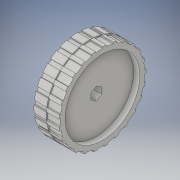
# Autodesk Inventor part: WheelV2
Saved by Autodesk Inventor 2019 (Build 230136000, 136)
## iProperties
Created: 2021-09-16
Part Number: WheelV2
Material: Generic
Document SubType Name: Modeling
Designer: timmy
Density: 1 g/cm^3
Appearance: Default
Author: timmy
Autodesk Inventor part; units mm, degrees
ref_plane "YZ Plane" through (0, 0, 0) normal (1, 0, 0) x (0, 1, 0)
ref_plane "XZ Plane" through (0, 0, 0) normal (0, 1, 0) x (-1, 0, 0)
sketch "Sketch1" plane through (0, 0, 0) normal (1, 0, 0) x (0, 1, 0)
  circle A0 centre (0, 0) radius 83.82
  circle A1 centre (0, 0) radius 86.36 construction
  line L0 (86.36, 0) -> (86.0238, -7.6126)
  line L1 (86.0238, -7.6126) -> (88.5638, -7.7247)
  line L2 (86.36, 0) -> (88.9, 0)
  line L3 (83.6468, 21.4769) -> (86.107, 22.1085)
  line L4 (83.6468, 21.4769) -> (85.2144, 14.0198)
  line L5 (85.2144, 14.0198) -> (87.7024, 14.5429)
  line L6 (75.6778, 41.6042) -> (77.9037, 42.8279)
  line L7 (75.6778, 41.6042) -> (79.0506, 34.7713)
  line L8 (79.0506, 34.7713) -> (81.3304, 35.8967)
  line L9 (62.9537, 59.1175) -> (64.8053, 60.8562)
  line L10 (62.9537, 59.1175) -> (67.9198, 53.338)
  line L11 (67.9198, 53.338) -> (69.8481, 54.995)
  line L12 (46.274, 72.9162) -> (47.635, 75.0608)
  line L13 (46.274, 72.9162) -> (52.5214, 68.5533)
  line L14 (52.5214, 68.5533) -> (53.9771, 70.6377)
  line L15 (26.6867, 82.1332) -> (27.4716, 84.5489)
  line L16 (26.6867, 82.1332) -> (33.8228, 79.4611)
  line L17 (33.8228, 79.4611) -> (34.7144, 81.8421)
  line L18 (5.4226, 86.1896) -> (5.5821, 88.7246)
  line L19 (5.4226, 86.1896) -> (12.999, 85.3761)
  line L20 (12.999, 85.3761) -> (13.2705, 87.904)
  line L21 (-16.1823, 84.8303) -> (-16.6582, 87.3253)
  line L22 (-16.1823, 84.8303) -> (-8.6415, 85.9266)
  line L23 (-8.6415, 85.9266) -> (-9.0073, 88.4425)
  line L24 (-36.7703, 78.1409) -> (-37.8518, 80.4391)
  line L25 (-36.7703, 78.1409) -> (-29.7391, 81.078)
  line L26 (-29.7391, 81.078) -> (-30.7191, 83.4239)
  line L27 (-55.0479, 66.5415) -> (-56.667, 68.4986)
  line L28 (-55.0479, 66.5415) -> (-48.9681, 71.1349)
  line L29 (-48.9681, 71.1349) -> (-50.5006, 73.1635)
  line L30 (-69.8667, 50.7611) -> (-71.9216, 52.2541)
  line L31 (-69.8667, 50.7611) -> (-65.1202, 56.7222)
  line L32 (-65.1202, 56.7222) -> (-67.1091, 58.3059)
  line L33 (-80.2955, 31.7912) -> (-82.6571, 32.7263)
  line L34 (-80.2955, 31.7912) -> (-77.1806, 38.7455)
  line L35 (-77.1806, 38.7455) -> (-79.5008, 39.7848)
  line L36 (-85.679, 10.8238) -> (-88.199, 11.1421)
  line L37 (-85.679, 10.8238) -> (-84.3914, 18.3342)
  line L38 (-84.3914, 18.3342) -> (-86.8972, 18.7638)
  line L39 (-85.679, -10.8238) -> (-88.199, -11.1421)
  line L40 (-85.679, -10.8238) -> (-86.2996, -3.2291)
  line L41 (-86.2996, -3.2291) -> (-88.8336, -3.4361)
  line L42 (-80.2955, -31.7912) -> (-82.6571, -32.7263)
  line L43 (-80.2955, -31.7912) -> (-82.7853, -24.5895)
  line L44 (-82.7853, -24.5895) -> (-85.1882, -25.4202)
  line L45 (-69.8667, -50.7611) -> (-71.9216, -52.2541)
  line L46 (-69.8667, -50.7611) -> (-74.0693, -44.4048)
  line L47 (-74.0693, -44.4048) -> (-76.1901, -45.807)
  line L48 (-55.0479, -66.5415) -> (-56.667, -68.4986)
  line L49 (-55.0479, -66.5415) -> (-60.6992, -61.4301)
  line L50 (-60.6992, -61.4301) -> (-62.4047, -63.3156)
  line L51 (-36.7703, -78.1409) -> (-37.8518, -80.4391)
  line L52 (-36.7703, -78.1409) -> (-43.5152, -74.5954)
  line L53 (-43.5152, -74.5954) -> (-44.6982, -76.8458)
  line L54 (-16.1823, -84.8303) -> (-16.6582, -87.3253)
  line L55 (-16.1823, -84.8303) -> (-23.597, -83.0736)
  line L56 (-23.597, -83.0736) -> (-24.1831, -85.5476)
  line L57 (5.4226, -86.1896) -> (5.5821, -88.7246)
  line L58 (5.4226, -86.1896) -> (-2.1961, -86.3321)
  line L59 (-2.1961, -86.3321) -> (-2.1485, -88.874)
  line L60 (26.6867, -82.1332) -> (27.4716, -84.5489)
  line L61 (26.6867, -82.1332) -> (19.3428, -84.1659)
  line L62 (19.3428, -84.1659) -> (20.021, -86.6162)
  line L63 (46.274, -72.9162) -> (47.635, -75.0608)
  line L64 (46.274, -72.9162) -> (39.6664, -76.7113)
  line L65 (39.6664, -76.7113) -> (40.9326, -78.916)
  line L66 (62.9537, -59.1175) -> (64.8053, -60.8562)
  line L67 (62.9537, -59.1175) -> (57.4975, -64.4367)
  line L68 (57.4975, -64.4367) -> (59.2722, -66.2572)
  line L69 (75.6778, -41.6042) -> (77.9037, -42.8279)
  line L70 (75.6778, -41.6042) -> (71.7159, -48.1132)
  line L71 (71.7159, -48.1132) -> (73.8876, -49.4352)
  line L72 (83.6468, -21.4769) -> (86.107, -22.1085)
  line L73 (83.6468, -21.4769) -> (81.4281, -28.7667)
  line L74 (81.4281, -28.7667) -> (83.8603, -29.507)
  arc A2 (86.107, 22.1085) -> (81.3304, 35.8967) centre (0, 0) ccw
  arc A3 (88.9, 0) -> (87.7024, 14.5429) centre (0, 0) ccw
  arc A4 (86.107, -22.1085) -> (88.5638, -7.7247) centre (0, 0) ccw
  arc A5 (77.9037, -42.8279) -> (83.8603, -29.507) centre (0, 0) ccw
  arc A6 (64.8053, -60.8562) -> (73.8876, -49.4352) centre (0, 0) ccw
  arc A7 (47.635, -75.0608) -> (59.2722, -66.2572) centre (0, 0) ccw
  arc A8 (27.4716, -84.5489) -> (40.9326, -78.916) centre (0, 0) ccw
  arc A9 (77.9037, 42.8279) -> (69.8481, 54.995) centre (0, 0) ccw
  arc A10 (64.8053, 60.8562) -> (53.9771, 70.6377) centre (0, 0) ccw
  arc A11 (47.635, 75.0608) -> (34.7144, 81.8421) centre (0, 0) ccw
  arc A12 (27.4716, 84.5489) -> (13.2705, 87.904) centre (0, 0) ccw
  arc A13 (5.5821, 88.7246) -> (-9.0073, 88.4425) centre (0, 0) ccw
  arc A14 (-16.6582, 87.3253) -> (-30.7191, 83.4239) centre (0, 0) ccw
  arc A15 (-37.8518, 80.4391) -> (-50.5006, 73.1635) centre (0, 0) ccw
  arc A16 (-56.667, 68.4986) -> (-67.1091, 58.3059) centre (0, 0) ccw
  arc A17 (-71.9216, 52.2541) -> (-79.5008, 39.7848) centre (0, 0) ccw
  arc A18 (-82.6571, 32.7263) -> (-86.8972, 18.7638) centre (0, 0) ccw
  arc A19 (-88.199, 11.1421) -> (-88.8336, -3.4361) centre (0, 0) ccw
  arc A20 (-88.199, -11.1421) -> (-85.1882, -25.4202) centre (0, 0) ccw
  arc A21 (-82.6571, -32.7263) -> (-76.1901, -45.807) centre (0, 0) ccw
  arc A22 (-71.9216, -52.2541) -> (-62.4047, -63.3156) centre (0, 0) ccw
  arc A23 (-56.667, -68.4986) -> (-44.6982, -76.8458) centre (0, 0) ccw
  arc A24 (-37.8518, -80.4391) -> (-24.1831, -85.5476) centre (0, 0) ccw
  arc A25 (-16.6582, -87.3253) -> (-2.1485, -88.874) centre (0, 0) ccw
  arc A26 (5.5821, -88.7246) -> (20.021, -86.6162) centre (0, 0) ccw
  dimension "d14" = 7.62
  dimension "d17" = 360
  constraints: 150 end point, 50 point on circle, 26 centre point, 1 coincident, 1 horizontal, 1 perpendicular, 179 other
  measures "d14" distance of L0.start L0.end
extrude "Extrusion1" add sketch "Sketch1" along normal blind 50.8 contours A0 | L0 L1 A4 L72 L73 L74 A5 L69 L70 L71 A6 L66 L67 L68 A7 L63 L64 L65 A8 L60 L61 L62 A26 L57 L58 L59 A25 L54 L55 L56 A24 L51 L52 L53 A23 L48 L49 L50 A22 L45 L46 L47 A21 L42 L43 L44 A20 L39 L40 L41 A19 L36 L37 L38 A18 L33 L34 L35 A17 L30 L31 L32 A16 L27 L28 L29 A15 L24 L25 L26 A14 L21 L22 L23 A13 L18 L19 L20 A12 L15 L16 L17 A11 L12 L13 L14 A10 L9 L10 L11 A9 L6 L7 L8 A2 L3 L4 L5 A3 L2
sketch "Sketch2" plane through (50.8, 0, 0) normal (1, 0, 0) x (0, -0.3273, 0.9449)
  arc A0 (-7.296, -88.6001) -> (7.296, -88.6001) centre (0, 0) ccw projected
  circle A1 centre (0, 0) radius 76.2
  line L0 (-35.3524, -78.7925) -> (-28.2693, -81.6021) projected
  line L1 (-28.2693, -81.6021) -> (-29.1008, -84.0021) projected
  arc A2 (-29.1008, -84.0021) -> (-14.9671, -87.631) centre (0, 0) ccw projected
  line L2 (-14.9671, -87.631) -> (-14.6469, -85.1089) projected
  line L3 (-14.6469, -85.1089) -> (-7.0876, -86.0687) projected
  line L4 (-7.0876, -86.0687) -> (-7.296, -88.6001) projected
  line L5 (7.296, -88.6001) -> (6.979, -86.0775) projected
  line L6 (6.979, -86.0775) -> (14.5395, -85.1273) projected
  line L7 (14.5395, -85.1273) -> (14.9671, -87.631) projected
  arc A3 (14.9671, -87.631) -> (29.1008, -84.0021) centre (0, 0) ccw projected
  line L8 (29.1008, -84.0021) -> (28.1663, -81.6377) projected
  line L9 (28.1663, -81.6377) -> (35.253, -78.837) projected
  line L10 (35.253, -78.837) -> (36.2899, -81.1558) projected
  arc A4 (36.2899, -81.1558) -> (49.077, -74.126) centre (0, 0) ccw projected
  line L11 (49.077, -74.126) -> (47.5839, -72.0682) projected
  line L12 (47.5839, -72.0682) -> (53.7514, -67.5931) projected
  line L13 (53.7514, -67.5931) -> (55.3324, -69.5812) projected
  arc A5 (55.3324, -69.5812) -> (65.9695, -59.5922) centre (0, 0) ccw projected
  line L14 (65.9695, -59.5922) -> (64.0116, -57.9704) projected
  line L15 (64.0116, -57.9704) -> (68.8725, -52.1021) projected
  line L16 (68.8725, -52.1021) -> (70.8981, -53.6346) projected
  arc A6 (70.8981, -53.6346) -> (78.717, -41.3141) centre (0, 0) ccw projected
  line L17 (78.717, -41.3141) -> (76.4172, -40.2301) projected
  line L18 (76.4172, -40.2301) -> (79.666, -33.3374) projected
  line L19 (79.666, -33.3374) -> (82.0091, -34.3179) projected
  arc A7 (82.0091, -34.3179) -> (86.5183, -20.44) centre (0, 0) ccw projected
  line L20 (86.5183, -20.44) -> (84.0212, -19.962) projected
  line L21 (84.0212, -19.962) -> (85.4538, -12.4779) projected
  line L22 (85.4538, -12.4779) -> (87.9671, -12.8449) projected
  arc A8 (87.9671, -12.8449) -> (88.8834, 1.7184) centre (0, 0) ccw projected
  line L23 (88.8834, 1.7184) -> (86.3459, 1.5604) projected
  line L24 (86.3459, 1.5604) -> (85.8722, 9.1656) projected
  line L25 (85.8722, 9.1656) -> (88.3979, 9.4352) projected
  arc A9 (88.3979, 9.4352) -> (85.6636, 23.7688) centre (0, 0) ccw projected
  line L26 (85.6636, 23.7688) -> (83.2451, 22.9847) projected
  line L27 (83.2451, 22.9847) -> (80.895, 30.2332) projected
  line L28 (80.895, 30.2332) -> (83.2743, 31.1224) projected
  arc A10 (83.2743, 31.1224) -> (77.0613, 44.3257) centre (0, 0) ccw projected
  line L29 (77.0613, 44.3257) -> (74.9138, 42.9648) projected
  line L30 (74.9138, 42.9648) -> (70.8348, 49.4012) projected
  line L31 (70.8348, 49.4012) -> (72.9182, 50.8541) projected
  arc A11 (72.9182, 50.8541) -> (63.6169, 62.0975) centre (0, 0) ccw projected
  line L32 (63.6169, 62.0975) -> (61.8753, 60.2453) projected
  line L33 (61.8753, 60.2453) -> (56.3239, 65.465) projected
  line L34 (56.3239, 65.465) -> (57.9805, 67.3905) projected
  arc A12 (57.9805, 67.3905) -> (46.1752, 75.9675) centre (0, 0) ccw projected
  line L35 (46.1752, 75.9675) -> (44.949, 73.7403) projected
  line L36 (44.949, 73.7403) -> (38.2739, 77.4155) projected
  line L37 (38.2739, 77.4155) -> (39.3996, 79.6924) projected
  arc A13 (39.3996, 79.6924) -> (25.8322, 85.0641) centre (0, 0) ccw projected
  line L38 (25.8322, 85.0641) -> (25.1984, 82.602) projected
  line L39 (25.1984, 82.602) -> (17.819, 84.5017) projected
  line L40 (17.819, 84.5017) -> (18.343, 86.987) projected
  arc A14 (18.343, 86.987) -> (3.866, 88.8159) centre (0, 0) ccw projected
  line L41 (3.866, 88.8159) -> (3.8644, 86.2735) projected
  line L42 (3.8644, 86.2735) -> (-3.7556, 86.2783) projected
  line L43 (-3.7556, 86.2783) -> (-3.866, 88.8159) projected
  arc A15 (-3.866, 88.8159) -> (-18.343, 86.987) centre (0, 0) ccw projected
  line L44 (-18.343, 86.987) -> (-17.7123, 84.5241) projected
  line L45 (-17.7123, 84.5241) -> (-25.0941, 82.6337) projected
  line L46 (-25.0941, 82.6337) -> (-25.8322, 85.0641) projected
  arc A16 (-25.8322, 85.0641) -> (-39.3996, 79.6924) centre (0, 0) ccw projected
  line L47 (-39.3996, 79.6924) -> (-38.1762, 77.4637) projected
  line L48 (-38.1762, 77.4637) -> (-44.8559, 73.797) projected
  line L49 (-44.8559, 73.797) -> (-46.1752, 75.9675) projected
  arc A17 (-46.1752, 75.9675) -> (-57.9805, 67.3905) centre (0, 0) ccw projected
  line L50 (-57.9805, 67.3905) -> (-56.2412, 65.5361) projected
  line L51 (-56.2412, 65.5361) -> (-61.7993, 60.3233) projected
  line L52 (-61.7993, 60.3233) -> (-63.6169, 62.0975) projected
  arc A18 (-63.6169, 62.0975) -> (-72.9182, 50.8541) centre (0, 0) ccw projected
  line L53 (-72.9182, 50.8541) -> (-70.7725, 49.4905) projected
  line L54 (-70.7725, 49.4905) -> (-74.8595, 43.0593) projected
  line L55 (-74.8595, 43.0593) -> (-77.0613, 44.3257) projected
  arc A19 (-77.0613, 44.3257) -> (-83.2743, 31.1224) centre (0, 0) ccw projected
  line L56 (-83.2743, 31.1224) -> (-80.8568, 30.3353) projected
  line L57 (-80.8568, 30.3353) -> (-83.2161, 23.0897) projected
  line L58 (-83.2161, 23.0897) -> (-85.6636, 23.7688) projected
  arc A20 (-85.6636, 23.7688) -> (-88.3979, 9.4352) centre (0, 0) ccw projected
  line L59 (-88.3979, 9.4352) -> (-85.8606, 9.274) projected
  line L60 (-85.8606, 9.274) -> (-86.3439, 1.6693) projected
  line L61 (-86.3439, 1.6693) -> (-88.8834, 1.7184) projected
  arc A21 (-88.8834, 1.7184) -> (-87.9671, -12.8449) centre (0, 0) ccw projected
  line L62 (-87.9671, -12.8449) -> (-85.4695, -12.3701) projected
  line L63 (-85.4695, -12.3701) -> (-84.0464, -19.856) projected
  line L64 (-84.0464, -19.856) -> (-86.5183, -20.44) projected
  arc A22 (-86.5183, -20.44) -> (-82.0091, -34.3179) centre (0, 0) ccw projected
  line L65 (-82.0091, -34.3179) -> (-79.708, -33.2368) projected
  line L66 (-79.708, -33.2368) -> (-76.4679, -40.1337) projected
  line L67 (-76.4679, -40.1337) -> (-78.717, -41.3141) projected
  arc A23 (-78.717, -41.3141) -> (-70.8981, -53.6346) centre (0, 0) ccw projected
  line L68 (-70.8981, -53.6346) -> (-68.9381, -52.0152) projected
  line L69 (-68.9381, -52.0152) -> (-64.0847, -57.8896) projected
  line L70 (-64.0847, -57.8896) -> (-65.9695, -59.5922) projected
  arc A24 (-65.9695, -59.5922) -> (-55.3324, -69.5812) centre (0, 0) ccw projected
  line L71 (-55.3324, -69.5812) -> (-53.8367, -67.5253) projected
  line L72 (-53.8367, -67.5253) -> (-47.6748, -72.0081) projected
  line L73 (-47.6748, -72.0081) -> (-49.077, -74.126) projected
  arc A25 (-49.077, -74.126) -> (-36.2899, -81.1558) centre (0, 0) ccw projected
  line L74 (-36.2899, -81.1558) -> (-35.3524, -78.7925) projected
  dimension "d3" = 12.7
  constraints: 1 centre point
  measures "d3" radial gap between concentric circles of A0 A1
extrude "Extrusion2" cut sketch "Sketch2" against normal blind 12.7 contours A1
sketch "Sketch4" plane through (0, 0, 0) normal (-1, 0, 0) x (0, 0.3273, -0.9449)
  circle A0 centre (0, 0) radius 76.2 projected
extrude "Extrusion3" cut sketch "Sketch4" against normal blind 12.7
sketch "Sketch5" plane through (38.1, 0, 0) normal (1, 0, 0) x (0, 0, -1)
  line L0 (0, 0) -> (0, 12.7)
  line L1 (0, 12.7) -> (10.9985, 6.35)
  line L2 (10.9985, 6.35) -> (10.9985, -6.35)
  line L3 (10.9985, -6.35) -> (0, -12.7)
  line L4 (0, -12.7) -> (-10.9985, -6.35)
  line L5 (-10.9985, -6.35) -> (-10.9985, 6.35)
  line L6 (-10.9985, 6.35) -> (0, 12.7)
  dimension "d8" = 12.7
  constraints: 14 end point, 1 coincident, 1 vertical, 13 other
  measures "d8" distance of L0.start L0.end
extrude "Extrusion4" cut sketch "Sketch5" against normal blind 127
ref_plane "Work Plane1" through (25.4, 0, 0) normal (1, 0, 0) x (0, 0, -1)
sketch "Sketch6" plane through (25.4, 0, 0) normal (1, 0, 0) x (0, 0, -1)
  circle A0 centre (0, 0) radius 76.2 projected
  line L0 (7.6126, 86.0238) -> (0, 86.36) projected
  line L1 (0, 86.36) -> (0, 88.9) projected
  arc A1 (0, 88.9) -> (-14.5429, 87.7024) centre (0, 0) ccw projected
  line L2 (-14.5429, 87.7024) -> (-14.0198, 85.2144) projected
  line L3 (-14.0198, 85.2144) -> (-21.4769, 83.6468) projected
  line L4 (-21.4769, 83.6468) -> (-22.1085, 86.107) projected
  arc A2 (-22.1085, 86.107) -> (-35.8967, 81.3304) centre (0, 0) ccw projected
  line L5 (-35.8967, 81.3304) -> (-34.7713, 79.0506) projected
  line L6 (-34.7713, 79.0506) -> (-41.6042, 75.6778) projected
  line L7 (-41.6042, 75.6778) -> (-42.8279, 77.9037) projected
  arc A3 (-42.8279, 77.9037) -> (-54.995, 69.8481) centre (0, 0) ccw projected
  line L8 (-54.995, 69.8481) -> (-53.338, 67.9198) projected
  line L9 (-53.338, 67.9198) -> (-59.1175, 62.9537) projected
  line L10 (-59.1175, 62.9537) -> (-60.8562, 64.8053) projected
  arc A4 (-60.8562, 64.8053) -> (-70.6377, 53.9771) centre (0, 0) ccw projected
  line L11 (-70.6377, 53.9771) -> (-68.5533, 52.5214) projected
  line L12 (-68.5533, 52.5214) -> (-72.9162, 46.274) projected
  line L13 (-72.9162, 46.274) -> (-75.0608, 47.635) projected
  arc A5 (-75.0608, 47.635) -> (-81.8421, 34.7144) centre (0, 0) ccw projected
  line L14 (-81.8421, 34.7144) -> (-79.4611, 33.8228) projected
  line L15 (-79.4611, 33.8228) -> (-82.1332, 26.6867) projected
  line L16 (-82.1332, 26.6867) -> (-84.5489, 27.4716) projected
  arc A6 (-84.5489, 27.4716) -> (-87.904, 13.2705) centre (0, 0) ccw projected
  line L17 (-87.904, 13.2705) -> (-85.3761, 12.999) projected
  line L18 (-85.3761, 12.999) -> (-86.1896, 5.4226) projected
  line L19 (-86.1896, 5.4226) -> (-88.7246, 5.5821) projected
  arc A7 (-88.7246, 5.5821) -> (-88.4425, -9.0073) centre (0, 0) ccw projected
  line L20 (-88.4425, -9.0073) -> (-85.9266, -8.6415) projected
  line L21 (-85.9266, -8.6415) -> (-84.8303, -16.1823) projected
  line L22 (-84.8303, -16.1823) -> (-87.3253, -16.6582) projected
  arc A8 (-87.3253, -16.6582) -> (-83.4239, -30.7191) centre (0, 0) ccw projected
  line L23 (-83.4239, -30.7191) -> (-81.078, -29.7391) projected
  line L24 (-81.078, -29.7391) -> (-78.1409, -36.7703) projected
  line L25 (-78.1409, -36.7703) -> (-80.4391, -37.8518) projected
  arc A9 (-80.4391, -37.8518) -> (-73.1635, -50.5006) centre (0, 0) ccw projected
  line L26 (-73.1635, -50.5006) -> (-71.1349, -48.9681) projected
  line L27 (-71.1349, -48.9681) -> (-66.5415, -55.0479) projected
  line L28 (-66.5415, -55.0479) -> (-68.4986, -56.667) projected
  arc A10 (-68.4986, -56.667) -> (-58.3059, -67.1091) centre (0, 0) ccw projected
  line L29 (-58.3059, -67.1091) -> (-56.7222, -65.1202) projected
  line L30 (-56.7222, -65.1202) -> (-50.7611, -69.8667) projected
  line L31 (-50.7611, -69.8667) -> (-52.2541, -71.9216) projected
  arc A11 (-52.2541, -71.9216) -> (-39.7848, -79.5008) centre (0, 0) ccw projected
  line L32 (-39.7848, -79.5008) -> (-38.7455, -77.1806) projected
  line L33 (-38.7455, -77.1806) -> (-31.7912, -80.2955) projected
  line L34 (-31.7912, -80.2955) -> (-32.7263, -82.6571) projected
  arc A12 (-32.7263, -82.6571) -> (-18.7638, -86.8972) centre (0, 0) ccw projected
  line L35 (-18.7638, -86.8972) -> (-18.3342, -84.3914) projected
  line L36 (-18.3342, -84.3914) -> (-10.8238, -85.679) projected
  line L37 (-10.8238, -85.679) -> (-11.1421, -88.199) projected
  arc A13 (-11.1421, -88.199) -> (3.4361, -88.8336) centre (0, 0) ccw projected
  line L38 (3.4361, -88.8336) -> (3.2291, -86.2996) projected
  line L39 (3.2291, -86.2996) -> (10.8238, -85.679) projected
  line L40 (10.8238, -85.679) -> (11.1421, -88.199) projected
  arc A14 (11.1421, -88.199) -> (25.4202, -85.1882) centre (0, 0) ccw projected
  line L41 (25.4202, -85.1882) -> (24.5895, -82.7853) projected
  line L42 (24.5895, -82.7853) -> (31.7912, -80.2955) projected
  line L43 (31.7912, -80.2955) -> (32.7263, -82.6571) projected
  arc A15 (32.7263, -82.6571) -> (45.807, -76.1901) centre (0, 0) ccw projected
  line L44 (45.807, -76.1901) -> (44.4048, -74.0693) projected
  line L45 (44.4048, -74.0693) -> (50.7611, -69.8667) projected
  line L46 (50.7611, -69.8667) -> (52.2541, -71.9216) projected
  arc A16 (52.2541, -71.9216) -> (63.3156, -62.4047) centre (0, 0) ccw projected
  line L47 (63.3156, -62.4047) -> (61.4301, -60.6992) projected
  line L48 (61.4301, -60.6992) -> (66.5415, -55.0479) projected
  line L49 (66.5415, -55.0479) -> (68.4986, -56.667) projected
  arc A17 (68.4986, -56.667) -> (76.8458, -44.6982) centre (0, 0) ccw projected
  line L50 (76.8458, -44.6982) -> (74.5954, -43.5152) projected
  line L51 (74.5954, -43.5152) -> (78.1409, -36.7703) projected
  line L52 (78.1409, -36.7703) -> (80.4391, -37.8518) projected
  arc A18 (80.4391, -37.8518) -> (85.5476, -24.1831) centre (0, 0) ccw projected
  line L53 (85.5476, -24.1831) -> (83.0736, -23.597) projected
  line L54 (83.0736, -23.597) -> (84.8303, -16.1823) projected
  line L55 (84.8303, -16.1823) -> (87.3253, -16.6582) projected
  arc A19 (87.3253, -16.6582) -> (88.874, -2.1485) centre (0, 0) ccw projected
  line L56 (88.874, -2.1485) -> (86.3321, -2.1961) projected
  line L57 (86.3321, -2.1961) -> (86.1896, 5.4226) projected
  line L58 (86.1896, 5.4226) -> (88.7246, 5.5821) projected
  arc A20 (88.7246, 5.5821) -> (86.6162, 20.021) centre (0, 0) ccw projected
  line L59 (86.6162, 20.021) -> (84.1659, 19.3428) projected
  line L60 (84.1659, 19.3428) -> (82.1332, 26.6867) projected
  line L61 (82.1332, 26.6867) -> (84.5489, 27.4716) projected
  arc A21 (84.5489, 27.4716) -> (78.916, 40.9326) centre (0, 0) ccw projected
  line L62 (78.916, 40.9326) -> (76.7113, 39.6664) projected
  line L63 (76.7113, 39.6664) -> (72.9162, 46.274) projected
  line L64 (72.9162, 46.274) -> (75.0608, 47.635) projected
  arc A22 (75.0608, 47.635) -> (66.2572, 59.2722) centre (0, 0) ccw projected
  line L65 (66.2572, 59.2722) -> (64.4367, 57.4975) projected
  line L66 (64.4367, 57.4975) -> (59.1175, 62.9537) projected
  line L67 (59.1175, 62.9537) -> (60.8562, 64.8053) projected
  arc A23 (60.8562, 64.8053) -> (49.4352, 73.8876) centre (0, 0) ccw projected
  line L68 (49.4352, 73.8876) -> (48.1132, 71.7159) projected
  line L69 (48.1132, 71.7159) -> (41.6042, 75.6778) projected
  line L70 (41.6042, 75.6778) -> (42.8279, 77.9037) projected
  arc A24 (42.8279, 77.9037) -> (29.507, 83.8603) centre (0, 0) ccw projected
  line L71 (29.507, 83.8603) -> (28.7667, 81.4281) projected
  line L72 (28.7667, 81.4281) -> (21.4769, 83.6468) projected
  line L73 (21.4769, 83.6468) -> (22.1085, 86.107) projected
  arc A25 (22.1085, 86.107) -> (7.7247, 88.5638) centre (0, 0) ccw projected
  line L74 (7.7247, 88.5638) -> (7.6126, 86.0238) projected
  line L75 (-60.8562, 64.8053) -> (-59.1175, 62.9537) projected
  line L76 (-60.8562, 64.8053) -> (-54.995, 69.8481)
  line L77 (-35.8967, 81.3304) -> (-34.7713, 79.0506) projected
  line L78 (-42.8279, 77.9037) -> (-35.8967, 81.3304)
  line L79 (-35.8967, 81.3304) -> (-22.1085, 86.107)
  line L80 (-14.0198, 85.2144) -> (-14.5429, 87.7024) projected
  line L81 (-14.5429, 87.7024) -> (-22.1085, 86.107)
  line L82 (0, 88.9) -> (7.7247, 88.5638)
  line L83 (22.1085, 86.107) -> (29.507, 83.8603)
  line L84 (42.8279, 77.9037) -> (49.4352, 73.8876)
  line L85 (60.8562, 64.8053) -> (66.2572, 59.2722)
  line L86 (78.916, 40.9326) -> (75.0608, 47.635)
  line L87 (84.5489, 27.4716) -> (86.6162, 20.021)
  line L88 (88.874, -2.1485) -> (88.7246, 5.5821)
  line L89 (-75.0608, 47.635) -> (-70.6377, 53.9771)
  line L90 (-84.5489, 27.4716) -> (-81.8421, 34.7144)
  line L91 (-87.904, 13.2705) -> (-85.3761, 12.999) projected
  line L92 (-88.7246, 5.5821) -> (-87.904, 13.2705)
  arc A26 (-84.5489, 27.4716) -> (-87.904, 13.2705) centre (0, 0) ccw projected
  arc A27 (-87.3253, -16.6582) -> (-83.4239, -30.7191) centre (0, 0) ccw projected
  line L93 (-87.3253, -16.6582) -> (-88.4425, -9.0073)
  line L94 (-83.4239, -30.7191) -> (-80.4391, -37.8518)
  arc A28 (-68.4986, -56.667) -> (-58.3059, -67.1091) centre (0, 0) ccw projected
  line L95 (-73.1635, -50.5006) -> (-68.4986, -56.667)
  line L96 (-58.3059, -67.1091) -> (-52.2541, -71.9216)
  arc A29 (-52.2541, -71.9216) -> (-39.7848, -79.5008) centre (0, 0) ccw projected
  line L97 (-39.7848, -79.5008) -> (-32.7263, -82.6571)
  line L98 (-18.7638, -86.8972) -> (-11.1421, -88.199)
  line L99 (3.4361, -88.8336) -> (11.1421, -88.199)
  line L100 (25.4202, -85.1882) -> (32.7263, -82.6571)
  line L101 (52.2541, -71.9216) -> (45.807, -76.1901)
  line L102 (63.3156, -62.4047) -> (68.4986, -56.667)
  line L103 (80.4391, -37.8518) -> (76.8458, -44.6982)
  line L104 (87.3253, -16.6582) -> (85.5476, -24.1831)
  constraints: 52 end point
extrude "Extrusion5" add sketch "Sketch6" along normal up to surface (25.4 mm away) contours L0 L1 L82 L74 | L83 L71 L72 L73 | L2 L3 L4 L81 | L84 L68 L69 L70 | L5 L6 L7 L78 | L85 L65 L66 L67 | L8 L9 L10 L76 | L86 L62 L63 L64 | L11 L12 L13 L89 | L87 L59 L60 L61 | L14 L15 L16 L90 | L88 L56 L57 L58 | L17 L18 L19 L92 | L104 L53 L54 L55 | L20 L21 L22 L93 | L103 L50 L51 L52 | L23 L24 L25 L94 | L102 L47 L48 L49 | L26 L27 L28 L95 | L101 L44 L45 L46 | L29 L30 L31 L96 | L100 L41 L42 L43 | L32 L33 L34 L97 | L99 L38 L39 L40 | L35 L36 L37 L98
sketch "Sketch7" plane through (50.8, 0, 0) normal (1, 0, 0) x (0, 0, -1)
  line L0 (22.1085, 86.107) -> (29.507, 83.8603) projected
  line L1 (0, 88.9) -> (7.7247, 88.5638) projected
  line L2 (-75.0608, 47.635) -> (-70.6377, 53.9771) projected
  line L3 (-84.5489, 27.4716) -> (-81.8421, 34.7144) projected
  line L4 (-88.7246, 5.5821) -> (-87.904, 13.2705) projected
  line L5 (-87.3253, -16.6582) -> (-88.4425, -9.0073) projected
  line L6 (-80.4391, -37.8518) -> (-83.4239, -30.7191) projected
  line L7 (42.8279, 77.9037) -> (49.4352, 73.8876) projected
  line L8 (60.8562, 64.8053) -> (66.2572, 59.2722) projected
  line L9 (75.0608, 47.635) -> (78.916, 40.9326) projected
  line L10 (84.5489, 27.4716) -> (86.6162, 20.021) projected
  line L11 (88.7246, 5.5821) -> (88.874, -2.1485) projected
  line L12 (87.3253, -16.6582) -> (85.5476, -24.1831) projected
  line L13 (80.4391, -37.8518) -> (76.8458, -44.6982) projected
  line L14 (68.4986, -56.667) -> (63.3156, -62.4047) projected
  line L15 (52.2541, -71.9216) -> (45.807, -76.1901) projected
  line L16 (32.7263, -82.6571) -> (25.4202, -85.1882) projected
  line L17 (-52.2541, -71.9216) -> (-58.3059, -67.1091) projected
  line L18 (-11.1421, -88.199) -> (-18.7638, -86.8972) projected
  line L19 (-68.4986, -56.667) -> (-73.1635, -50.5006) projected
  line L20 (-32.7263, -82.6571) -> (-39.7848, -79.5008) projected
  line L21 (11.1421, -88.199) -> (3.4361, -88.8336) projected
  line L22 (-35.8967, 81.3304) -> (-34.771, 79.0535)
  circle A0 centre (0, 0) radius 76.2 projected
  circle A1 centre (0, 0) radius 86.3625 construction
  line L23 (-22.1085, 86.107) -> (-21.4769, 83.6468)
  line L24 (-34.771, 79.0535) -> (-21.4769, 83.6468)
  arc A2 (-22.1085, 86.107) -> (-35.8967, 81.3304) centre (0, 0) ccw projected
  arc A3 (-22.1085, 86.107) -> (-35.8967, 81.3304) centre (0, 0) ccw
  arc A4 (-42.8279, 77.9037) -> (-54.995, 69.8481) centre (0, 0) ccw
  line L25 (-42.8279, 77.9037) -> (-41.6042, 75.6778)
  line L26 (-53.3384, 67.9227) -> (-41.6042, 75.6778)
  line L27 (-54.995, 69.8481) -> (-53.3384, 67.9227)
  arc A5 (-60.8562, 64.8053) -> (-70.6377, 53.9771) centre (0, 0) ccw
  line L28 (-60.8562, 64.8053) -> (-59.1175, 62.9537)
  line L29 (-68.5543, 52.5241) -> (-59.1175, 62.9537)
  line L30 (-70.6377, 53.9771) -> (-68.5543, 52.5241)
  arc A6 (-75.0608, 47.635) -> (-81.8421, 34.7144) centre (0, 0) ccw
  line L31 (-75.0608, 47.635) -> (-72.9162, 46.274)
  line L32 (-79.4628, 33.8252) -> (-72.9162, 46.274)
  line L33 (-81.8421, 34.7144) -> (-79.4628, 33.8252)
  arc A7 (-84.5489, 27.4716) -> (-87.904, 13.2705) centre (0, 0) ccw
  line L34 (-84.5489, 27.4716) -> (-82.1332, 26.6867)
  line L35 (-85.3783, 13.0009) -> (-82.1332, 26.6867)
  line L36 (-87.904, 13.2705) -> (-85.3783, 13.0009)
  arc A8 (-88.7246, 5.5821) -> (-88.4425, -9.0073) centre (0, 0) ccw
  line L37 (-88.7246, 5.5821) -> (-86.1896, 5.4226)
  line L38 (-85.9292, -8.6403) -> (-86.1896, 5.4226)
  line L39 (-88.4425, -9.0073) -> (-85.9292, -8.6403)
  arc A9 (-87.3253, -16.6582) -> (-83.4239, -30.7191) centre (0, 0) ccw
  line L40 (-87.3253, -16.6582) -> (-84.8303, -16.1823)
  line L41 (-81.0808, -29.7385) -> (-84.8303, -16.1823)
  line L42 (-83.4239, -30.7191) -> (-81.0808, -29.7385)
  arc A10 (-80.4391, -37.8518) -> (-73.1635, -50.5006) centre (0, 0) ccw
  line L43 (-80.4391, -37.8518) -> (-78.1409, -36.7703)
  line L44 (-71.1378, -48.9682) -> (-78.1409, -36.7703)
  line L45 (-73.1635, -50.5006) -> (-71.1378, -48.9682)
  arc A11 (-68.4986, -56.667) -> (-58.3059, -67.1091) centre (0, 0) ccw
  line L46 (-68.4986, -56.667) -> (-66.5415, -55.0479)
  line L47 (-56.725, -65.1211) -> (-66.5415, -55.0479)
  line L48 (-58.3059, -67.1091) -> (-56.725, -65.1211)
  arc A12 (-52.2541, -71.9216) -> (-39.7848, -79.5008) centre (0, 0) ccw
  line L49 (-52.2541, -71.9216) -> (-50.7611, -69.8667)
  line L50 (-38.7479, -77.1821) -> (-50.7611, -69.8667)
  line L51 (-39.7848, -79.5008) -> (-38.7479, -77.1821)
  arc A13 (-32.7263, -82.6571) -> (-18.7638, -86.8972) centre (0, 0) ccw
  line L52 (-32.7263, -82.6571) -> (-31.7912, -80.2955)
  line L53 (-18.3362, -84.3935) -> (-31.7912, -80.2955)
  line L54 (-18.7638, -86.8972) -> (-18.3362, -84.3935)
  arc A14 (-11.1421, -88.199) -> (3.4361, -88.8336) centre (0, 0) ccw
  line L55 (-11.1421, -88.199) -> (-10.8238, -85.679)
  line L56 (3.2277, -86.3021) -> (-10.8238, -85.679)
  line L57 (3.4361, -88.8336) -> (3.2277, -86.3021)
  arc A15 (11.1421, -88.199) -> (25.4202, -85.1882) centre (0, 0) ccw
  line L58 (11.1421, -88.199) -> (10.8238, -85.679)
  line L59 (24.5888, -82.7881) -> (10.8238, -85.679)
  line L60 (25.4202, -85.1882) -> (24.5888, -82.7881)
  arc A16 (32.7263, -82.6571) -> (45.807, -76.1901) centre (0, 0) ccw
  line L61 (32.7263, -82.6571) -> (31.7912, -80.2955)
  line L62 (44.4048, -74.0722) -> (31.7912, -80.2955)
  line L63 (45.807, -76.1901) -> (44.4048, -74.0722)
  arc A17 (52.2541, -71.9216) -> (63.3156, -62.4047) centre (0, 0) ccw
  line L64 (52.2541, -71.9216) -> (50.7611, -69.8667)
  line L65 (61.4308, -60.702) -> (50.7611, -69.8667)
  line L66 (63.3156, -62.4047) -> (61.4308, -60.702)
  arc A18 (68.4986, -56.667) -> (76.8458, -44.6982) centre (0, 0) ccw
  line L67 (68.4986, -56.667) -> (66.5415, -55.0479)
  line L68 (74.5968, -43.5178) -> (66.5415, -55.0479)
  line L69 (76.8458, -44.6982) -> (74.5968, -43.5178)
  arc A19 (80.4391, -37.8518) -> (85.5476, -24.1831) centre (0, 0) ccw
  line L70 (80.4391, -37.8518) -> (78.1409, -36.7703)
  line L71 (83.0756, -23.5991) -> (78.1409, -36.7703)
  line L72 (85.5476, -24.1831) -> (83.0756, -23.5991)
  arc A20 (87.3253, -16.6582) -> (88.874, -2.1485) centre (0, 0) ccw
  line L73 (87.3253, -16.6582) -> (84.8303, -16.1823)
  line L74 (86.3345, -2.1976) -> (84.8303, -16.1823)
  line L75 (88.874, -2.1485) -> (86.3345, -2.1976)
  arc A21 (88.7246, 5.5821) -> (86.6162, 20.021) centre (0, 0) ccw
  line L76 (88.7246, 5.5821) -> (86.1896, 5.4226)
  line L77 (84.1687, 19.3419) -> (86.1896, 5.4226)
  line L78 (86.6162, 20.021) -> (84.1687, 19.3419)
  arc A22 (84.5489, 27.4716) -> (78.916, 40.9326) centre (0, 0) ccw
  line L79 (84.5489, 27.4716) -> (82.1332, 26.6867)
  line L80 (76.7142, 39.6662) -> (82.1332, 26.6867)
  line L81 (78.916, 40.9326) -> (76.7142, 39.6662)
  arc A23 (75.0608, 47.635) -> (66.2572, 59.2722) centre (0, 0) ccw
  line L82 (75.0608, 47.635) -> (72.9162, 46.274)
  line L83 (64.4395, 57.498) -> (72.9162, 46.274)
  line L84 (66.2572, 59.2722) -> (64.4395, 57.498)
  arc A24 (60.8562, 64.8053) -> (49.4352, 73.8876) centre (0, 0) ccw
  line L85 (60.8562, 64.8053) -> (59.1175, 62.9537)
  line L86 (48.1159, 71.7171) -> (59.1175, 62.9537)
  line L87 (49.4352, 73.8876) -> (48.1159, 71.7171)
  arc A25 (42.8279, 77.9037) -> (29.507, 83.8603) centre (0, 0) ccw
  line L88 (42.8279, 77.9037) -> (41.6042, 75.6778)
  line L89 (28.7689, 81.4299) -> (41.6042, 75.6778)
  line L90 (29.507, 83.8603) -> (28.7689, 81.4299)
  arc A26 (22.1085, 86.107) -> (7.7247, 88.5638) centre (0, 0) ccw
  line L91 (22.1085, 86.107) -> (21.4769, 83.6468)
  line L92 (7.6143, 86.0262) -> (21.4769, 83.6468)
  line L93 (7.7247, 88.5638) -> (7.6143, 86.0262)
  arc A27 (0, 88.9) -> (-14.5429, 87.7024) centre (0, 0) ccw
  line L94 (0, 88.9) -> (0, 86.36)
  line L95 (-14.0188, 85.2171) -> (0, 86.36)
  line L96 (-14.5429, 87.7024) -> (-14.0188, 85.2171)
  dimension "d24" = 360
  constraints: 150 end point, 50 point on circle, 26 centre point, 2 coincident, 224 other
extrude "Extrusion6" cut sketch "Sketch7" against normal blind 25.4 contours A5 L28 L29 L30 | A6 L31 L32 L33 | A7 L34 L35 L36 | A8 L37 L38 L39 | A9 L40 L41 L42 | A10 L43 L44 L45 | A11 L46 L47 L48 | A12 L49 L50 L51 | A13 L52 L53 L54 | A14 L55 L56 L57 | A15 L58 L59 L60 | A16 L61 L62 L63 | A17 L64 L65 L66 | A18 L67 L68 L69 | A19 L70 L71 L72 | A20 L73 L74 L75 | A21 L76 L77 L78 | A22 L79 L80 L81 | A23 L82 L83 L84 | A24 L85 L86 L87 | A25 L88 L89 L90 | L91 L92 L93 A26 | L94 L95 L96 A27 | A2 L23 L24 L22 | L25 L26 L27 A4
body "Solid1"
